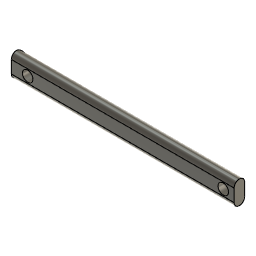
Sabrinica (Autodesk Fusion 360 design; units mm, degrees)
Autodesk Fusion 360 part; units mm, degrees
sketch "Sketch1" plane through (1.7731, -80, 44.5975) normal (0, -1, 0) x (1, 0, 0)
  circle A0 centre (-18.2269, 40.4025) radius 1
  line L0 (-21.3196, -42.597) -> (-21.3196, 42.597)
  line L1 (93.2269, 42.5973) -> (-81.7731, 42.5973)
  circle A1 centre (18.7731, 40.4025) radius 1
  line L2 (21.3196, -42.597) -> (21.3196, 42.597)
  line L3 (-21.3196, 42.597) -> (20.8249, 42.597)
  line L4 (20.8249, 42.597) -> (20.8249, 38.2081)
  line L5 (20.8249, 38.2081) -> (-21.3196, 38.2081)
  line L6 (-21.3196, 38.2081) -> (-21.3196, 42.597)
  line L7 (-21.3196, 42.597) -> (20.8249, 38.2081) construction
  line L8 (20.8249, 42.597) -> (-21.3196, 38.2081) construction
  point P0 (-0.2473, 40.4025)
  constraint horizontal L3
  constraint perpendicular L3 L4
  constraint parallel L3 L5
  constraint parallel L4 L6
  constraint coincident L0.end L3.start
  constraint coincident L7 P0
  constraint coincident L8 P0
extrude "Extrude1" add sketch "Sketch1" along normal blind 2
fillet "Fillet1" radius 1 4 edges at (1.5258, -80, 87.1945) (-19.5465, -80, 85) (1.5258, -80, 82.8055) (22.598, -80, 85)
delete_face "DeleteFace1" 1 faces at (21.938, -80.0596, 84.5216)
fillet "Fillet2" radius 1 2 edges at (1.5258, -82, 87.1945) (1.5258, -82, 82.8055)
